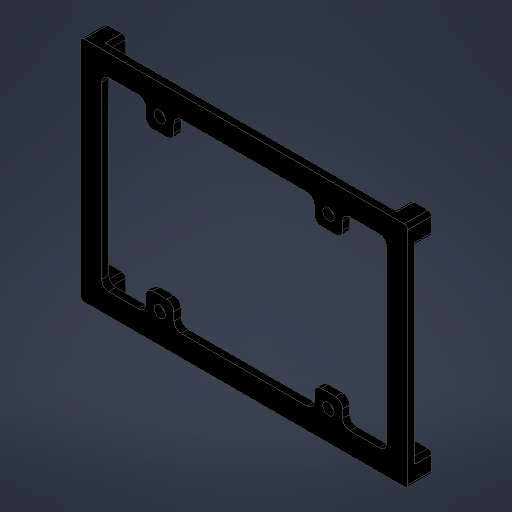
# Autodesk Inventor part: Jetson Adapter
Saved by Autodesk Inventor 2026.1 (Build 301233020, 233B)
## iProperties
Created: 2025-11-27
Part Number: Jetson Adapter
Material: Generic
Document SubType Name: Modeling
Designer: Bahaa
Density: 1 g/cm^3
Appearance: Default
Author: Bahaa
Autodesk Inventor part; units mm, degrees
ref_plane "YZ Plane" through (0, 0, 0) normal (1, 0, 0) x (0, 1, 0)
ref_plane "XZ Plane" through (0, 0, 0) normal (0, 1, 0) x (-1, 0, 0)
ref_plane "XY Plane" through (0, 0, 0) normal (0, 0, 1) x (1, 0, 0)
sketch "Sketch1" plane through (0, 0, 0) normal (0, 1, 0) x (-1, 0, 0)
  circle A0 centre (23.6881, 23.6881) radius 1.6
  line L0 (0, 0) -> (50, 0) construction
  line L1 (0, 0) -> (0, -50) construction
  circle A1 centre (23.6881, -23.6881) radius 1.6
  circle A2 centre (-23.6881, 23.6881) radius 1.6
  circle A3 centre (-23.6881, -23.6881) radius 1.6
  line L2 (-43, 29) -> (43, 29) construction
  line L3 (43, 29) -> (43, -29) construction
  line L4 (43, -29) -> (-43, -29) construction
  line L5 (-43, -29) -> (-43, 29) construction
  line L6 (-43, 29) -> (43, -29) construction
  line L7 (43, 29) -> (-43, -29) construction
  line L8 (-46, 32) -> (46, 32)
  line L9 (46, 32) -> (46, -32)
  line L10 (46, -32) -> (-46, -32)
  line L11 (-46, -32) -> (-46, 32)
  line L12 (-46, 32) -> (46, -32) construction
  line L13 (46, 32) -> (-46, -32) construction
  line L14 (40, 26) -> (46, 26)
  line L15 (46, 26) -> (46, 32)
  line L16 (46, 32) -> (40, 32)
  line L17 (40, 32) -> (40, 26)
  line L18 (40, 26) -> (46, 32) construction
  line L19 (46, 26) -> (40, 32) construction
  line L20 (-40, 26) -> (-46, 26)
  line L21 (-46, 26) -> (-46, 32)
  line L22 (-46, 32) -> (-40, 32)
  line L23 (-40, 32) -> (-40, 26)
  line L24 (-40, 26) -> (-46, 32) construction
  line L25 (-46, 26) -> (-40, 32) construction
  line L26 (-40, -26) -> (-46, -26)
  line L27 (-46, -26) -> (-46, -32)
  line L28 (-46, -32) -> (-40, -32)
  line L29 (-40, -32) -> (-40, -26)
  line L30 (-40, -26) -> (-46, -32) construction
  line L31 (-46, -26) -> (-40, -32) construction
  line L32 (40, -26) -> (46, -26)
  line L33 (46, -26) -> (46, -32)
  line L34 (46, -32) -> (40, -32)
  line L35 (40, -32) -> (40, -26)
  line L36 (40, -26) -> (46, -32) construction
  line L37 (46, -26) -> (40, -32) construction
  line L38 (-40, -26) -> (40, -26)
  line L39 (40, -26) -> (40, 26)
  line L40 (40, 26) -> (-40, 26)
  line L41 (-40, 26) -> (-40, -26)
  line L42 (-40, -26) -> (40, 26) construction
  line L43 (40, -26) -> (-40, 26) construction
  line L44 (19.6881, 27.6881) -> (27.6881, 27.6881)
  line L45 (27.6881, 27.6881) -> (27.6881, 19.6881)
  line L46 (27.6881, 19.6881) -> (19.6881, 19.6881)
  line L47 (19.6881, 19.6881) -> (19.6881, 27.6881)
  line L48 (19.6881, 27.6881) -> (27.6881, 19.6881) construction
  line L49 (27.6881, 27.6881) -> (19.6881, 19.6881) construction
  line L50 (19.6881, -19.6881) -> (27.6881, -19.6881)
  line L51 (27.6881, -19.6881) -> (27.6881, -27.6881)
  line L52 (27.6881, -27.6881) -> (19.6881, -27.6881)
  line L53 (19.6881, -27.6881) -> (19.6881, -19.6881)
  line L54 (19.6881, -19.6881) -> (27.6881, -27.6881) construction
  line L55 (27.6881, -19.6881) -> (19.6881, -27.6881) construction
  line L56 (-27.6881, -19.6881) -> (-19.6881, -19.6881)
  line L57 (-19.6881, -19.6881) -> (-19.6881, -27.6881)
  line L58 (-19.6881, -27.6881) -> (-27.6881, -27.6881)
  line L59 (-27.6881, -27.6881) -> (-27.6881, -19.6881)
  line L60 (-27.6881, -19.6881) -> (-19.6881, -27.6881) construction
  line L61 (-19.6881, -19.6881) -> (-27.6881, -27.6881) construction
  line L62 (-27.6881, 27.6881) -> (-19.6881, 27.6881)
  line L63 (-19.6881, 27.6881) -> (-19.6881, 19.6881)
  line L64 (-19.6881, 19.6881) -> (-27.6881, 19.6881)
  line L65 (-27.6881, 19.6881) -> (-27.6881, 27.6881)
  line L66 (-27.6881, 27.6881) -> (-19.6881, 19.6881) construction
  line L67 (-19.6881, 27.6881) -> (-27.6881, 19.6881) construction
  point P0 (27.6881, -26)
  point P1 (19.6881, -26)
  point P2 (-19.6881, -26)
  point P3 (-27.6881, -26)
  point P4 (-27.6881, 26)
  point P5 (-19.6881, 26)
  point P6 (19.6881, 26)
  point P7 (27.6881, 26)
  dimension "d0" = 3.2
  dimension "d5" = 23.6881
  dimension "d6" = 23.6881
  dimension "d7" = 50
  dimension "d8" = 50
  dimension "d9" = 86
  dimension "d10" = 58
  dimension "d11" = 92
  dimension "d12" = 64
  dimension "d13" = 8
  dimension "d14" = 8
  dimension "d15" = 8
  dimension "d16" = 8
  dimension "d17" = 8
  dimension "d18" = 8
  dimension "d19" = 8
  dimension "d20" = 8
  constraints: 136 end point, 22 midpoint, 22 parallel, 12 horizontal, 11 perpendicular, 4 centre point, 4 coincident, 3 symmetric about line, 1 vertical, 3 other
  measures "d0" diameter of A0
  measures "d5" horizontal distance of L0.start A0.centre
  measures "d6" horizontal distance of L0.start A0.centre
  measures "d7" distance of L0.start L0.end
  measures "d8" distance of L0.start L1.end
  measures "d9" distance of L3.end L4.end
  measures "d10" distance of L2.end L3.end
  measures "d11" distance of L9.end L10.end
  measures "d12" distance of L8.end L9.end
  measures "d13" distance of L45.end L46.end
  measures "d14" distance of L44.end L45.end
  measures "d15" distance of L51.end L52.end
  measures "d16" distance of L50.end L51.end
  measures "d17" distance of L57.end L58.end
  measures "d18" distance of L56.end L57.end
  measures "d19" distance of L63.end L64.end
  measures "d20" distance of L62.end L63.end
extrude "Extrusion1" add sketch "Sketch1" along normal blind 2 contours L8 L23 L20 L11 | L8 L17 L40 L45 L44 L47 L63 L62 L65 L23 | L20 L41 L26 L11 | L8 L9 L14 L17 | L26 L29 L10 L11 | L14 L9 L32 L39 | L65 L62 L63 L40 | L40 L63 L64 L65 | L38 L59 L58 L57 L53 L52 L51 L35 L10 L29 | L32 L9 L10 L35 | L45 L46 L47 L40 | L40 L47 L44 L45 | L59 L56 L57 L38 | L38 L57 L58 L59 | L51 L52 L53 L38 | L38 L53 L50 L51
extrude "Extrusion2" add sketch "Sketch1" along normal blind 4.7 from surface at 2 contours L8 L23 L20 L11 | L8 L9 L14 L17 | L26 L29 L10 L11 | L32 L9 L10 L35
sketch "Sketch2" plane through (-46, 6.7, 26) normal (0, 1, 0) x (1, 0, 0)
  point P0 (46, 26)
  point P1 (3, -3)
  point P2 (3, 55)
  point P3 (89, 55)
  point P4 (89, -3)
hole "Hole1" at (-43, 6.7, 29) at (-43, 6.7, -29) at (43, 6.7, 29) at (43, 6.7, -29) direction (0, -1, 0) diameter 3.9 depth 5.7
fillet "Fillet1" radius 2 20 edges at (40, 1, -26) (27.6881, 1, -26) (27.6881, 1, -19.6881) (19.6881, 1, -19.6881) (19.6881, 1, -26) (-19.6881, 1, -26) (-19.6881, 1, -19.6881) (-27.6881, 1, -19.6881) (-27.6881, 1, -26) (-40, 1, -26) (-40, 1, 26) (40, 1, 26) (27.6881, 1, 26) (27.6881, 1, 19.6881) (19.6881, 1, 26) (19.6881, 1, 19.6881) (-19.6881, 1, 26) (-19.6881, 1, 19.6881) (-27.6881, 1, 19.6881) (-27.6881, 1, 26)
fillet "Fillet2" radius 1 16 edges at (-40, 4.35, -26) (-40, 4.35, -32) (-46, 3.35, -32) (-46, 4.35, -26) (-40, 4.35, 26) (-46, 4.35, 26) (-40, 4.35, 32) (-46, 3.35, 32) (46, 4.35, 26) (40, 4.35, 26) (46, 3.35, 32) (40, 4.35, 32) (46, 3.35, -32) (46, 4.35, -26) (40, 4.35, -32) (40, 4.35, -26)
body "Solid1"
